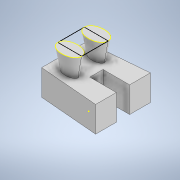
# Autodesk Inventor part: AutoPerson
Saved by Autodesk Inventor 2020 (Build 240168000, 168)
## iProperties
Created: 2020-02-07
Part Number: AutoPerson
Material: Generic
Document SubType Name: Modeling
Designer: cks4a449
Density: 1 g/cm^3
Appearance: Default
Author: cks4a449
Autodesk Inventor part; units mm, degrees
ref_plane "YZ Plane" through (0, 0, 0) normal (1, 0, 0) x (0, 1, 0)
ref_plane "XZ Plane" through (0, 0, 0) normal (0, 1, 0) x (-1, 0, 0)
ref_plane "XY Plane" through (0, 0, 0) normal (0, 0, 1) x (1, 0, 0)
sketch "Sketch1" plane through (0, 0, 0) normal (0, 1, 0) x (-1, 0, 0)
  line L0 (25.1646, -10.8178) -> (25.1646, -24.5338)
  line L1 (7.1306, -15.6438) -> (15.2586, -15.6438)
  line L2 (15.2586, -15.6438) -> (15.2586, -19.7078)
  line L3 (15.2586, -19.7078) -> (7.1306, -19.7078)
  line L4 (7.1306, -26.0578) -> (7.1306, -19.7078)
  line L5 (7.1306, -15.6438) -> (7.1306, -9.2938)
  line L6 (7.1306, -9.2938) -> (25.1646, -10.8178)
  line L7 (7.1306, -26.0578) -> (25.1646, -24.5338)
  point P0 (0, 0)
  dimension "d0" = 13.716
  dimension "d1" = 4.064
  dimension "d2" = 6.35
  dimension "d3" = 6.35
  dimension "d4" = 18.034
  dimension "d6" = 1.524
  dimension "d7" = 8.128
  constraints: 16 end point, 3 parallel, 1 horizontal, 1 perpendicular, 1 point on line, 1 vertical
  measures "d0" distance of L0.start L0.end
  measures "d1" distance between parallel lines of L1 L3
  measures "d2" distance of L1.start L5.end
  measures "d3" distance of L4.start L3.end
  measures "d4" distance between parallel lines of L4 L0
  measures "d6" vertical distance of L4.start L0.end
  measures "d7" distance between parallel lines of L4 L2
extrude "Extrusion1" add sketch "Sketch1" along normal blind 7.874
sketch "Sketch2" plane through (0, 7.874, 0) normal (0, 1, 0) x (1, 0, 0)
  line L0 (-15.2586, 15.6438) -> (-15.2586, 19.7078) projected
  line L1 (-7.1306, 26.0578) -> (-25.1646, 24.5338) projected
  line L2 (-25.1646, 24.5338) -> (-25.1646, 10.8178) projected
  line L3 (-7.1306, 9.2938) -> (-7.1306, 15.6438) projected
  ellipse E0 centre (-19.4146, 21.7325) end of major axis (-16.8746, 21.7325) minor radius 1.27
  ellipse E1 centre (-19.4146, 13.6192) end of major axis (-16.8746, 13.6192) minor radius 1.27
  line L4 (-15.2586, 19.7078) -> (-17.5953, 20.8462)
  line L5 (-21.2338, 22.6188) -> (-25.1646, 24.5338)
  line L6 (-25.1646, 19.7078) -> (-21.4913, 21.0013)
  line L7 (-17.3378, 22.4638) -> (-7.1306, 26.0578)
  line L8 (-15.2586, 15.6438) -> (-17.5953, 14.5054)
  line L9 (-21.2338, 12.7329) -> (-25.1646, 10.8178)
  line L10 (-25.1646, 15.6438) -> (-21.4913, 14.3504)
  line L11 (-17.3378, 12.8879) -> (-7.1306, 9.2938)
  point P0 (0, 0)
  dimension "d10" = 2.54
  dimension "d11" = 2.54
  dimension "d12" = 1.27
  dimension "d13" = 1.27
  constraints: 16 end point, 1 point on line, 22 other
extrude "Extrusion2" add sketch "Sketch2" along normal blind 6.35 draft 10 contours E1 | E0
sketch "Sketch8" plane through (0, 14.224, 0) normal (0, 1, 0) x (1, 0, 0)
  line L0 (-15.7549, 21.7325) -> (-15.7549, 13.6192)
  line L1 (-23.0742, 13.6192) -> (-23.0742, 21.7325)
  line L2 (-23.0742, 21.7325) -> (-15.7549, 21.7325)
  line L3 (-23.0742, 13.6192) -> (-15.7549, 13.6192)
  point P0 (0, 0)
  constraints: 8 end point, 2 horizontal alignment, 1 parallel, 1 perpendicular, 1 vertical, 2 other
body "Solid1"
